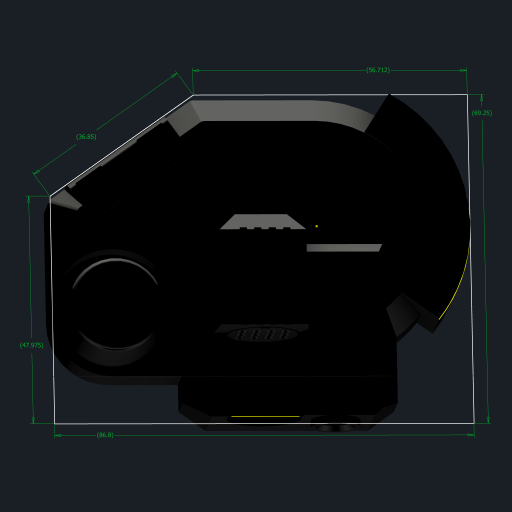
# Autodesk Inventor part: MidiController
Saved by Autodesk Inventor 2023 (Build 270158000, 158)
## iProperties
Created: 2023-06-16
Part Number: MidiController
Material: Generic
Document SubType Name: Modeling
Designer: valer
Density: 1 g/cm^3
Appearance: Default
Author: valer
Autodesk Inventor part; units mm, degrees
ref_plane "YZ Plane" through (0, 0, 0) normal (1, 0, 0) x (0, 1, 0)
ref_plane "XZ Plane" through (0, 0, 0) normal (0, 1, 0) x (-1, 0, 0)
ref_plane "XY Plane" through (0, 0, 0) normal (0, 0, 1) x (1, 0, 0)
sketch "Sketch1" plane through (0, 0, 0) normal (0, 0, 1) x (1, 0, 0)
  line L0 (-41.4, 33.875) -> (41.4, 33.875) construction
  line L1 (41.4, 33.875) -> (41.4, -33.875) construction
  line L2 (41.4, -33.875) -> (-41.4, -33.875) construction
  line L3 (-41.4, -33.875) -> (-41.4, 33.875) construction
  line L4 (-59.3343, 0) -> (66.206, 0) construction
  line L5 (0, -48.6206) -> (0, 54.5983) construction
  circle A0 centre (-28.595, -11.3999) radius 10.805 construction
  circle A1 centre (-28.595, -11.3999) radius 12.805
  line L6 (-28.595, -24.2049) -> (-14.35, -24.2049)
  line L7 (-14.35, -24.2049) -> (-14.35, -29.875)
  line L8 (-14.35, -29.875) -> (-8.85, -33.875)
  line L9 (-8.85, -33.875) -> (24.75, -33.875)
  line L10 (24.75, -33.875) -> (30.25, -29.875)
  line L11 (30.25, -29.875) -> (30.25, -16.055)
  line L12 (-14.35, -29.875) -> (30.25, -29.875) construction
  line L13 (-41.4, -11.3999) -> (-41.4, 12.6001)
  line L14 (-11.3118, 33.875) -> (-41.4, 12.6001)
  arc A2 (30.25, -16.055) -> (13.6882, 33.875) centre (13.6882, 6.1632) ccw
  line L15 (-11.3118, 33.875) -> (13.6882, 33.875)
  point P0 (0, 0)
  point P1 (-41.4, 0)
  point P2 (0, 33.875)
  dimension "d0" = 82.8
  dimension "d1" = 67.75
  dimension "d2" = 21.61
  dimension "d3" = 2
  dimension "d4" = 44.6
  dimension "d5" = 4
  dimension "d6" = 5.5
  dimension "d7" = 11.15
  dimension "d9" = 36.85
  dimension "d10" = 24
  dimension "d11" = 25
  dimension "d12" = 13.82
  constraints: 28 end point, 8 point on line, 5 tangent, 4 point on circle, 3 centre point, 3 perpendicular, 2 horizontal, 2 midpoint, 2 parallel, 1 coincident, 1 collinear, 1 equal length, 1 vertical
  measures "d0" distance of L0.start L0.end
  measures "d1" distance of L2.end L0.start
  measures "d2" diameter of A0
  measures "d3" radial gap between concentric circles of A1 A0
  measures "d4" distance between parallel lines of L11 L7
  measures "d5" distance between parallel lines of L9 L12
  measures "d6" horizontal distance of L7.end L8.end
  measures "d7" distance between parallel lines of L1 L11
  measures "d9" distance of L14.start L13.end
  measures "d10" distance of L13.start L13.end
  measures "d11" distance of L15.end L14.start
  measures "d12" distance of L10.end L11.end
extrude "Extrusion1" add sketch "Sketch1" along normal blind 9
sketch "Sketch2" plane through (0, 0, 9) normal (0, 0, 1) x (1, 0, 0)
  line L0 (-14.35, -29.875) -> (-8.85, -33.875) projected
  line L1 (-8.85, -33.875) -> (24.75, -33.875) projected
  line L2 (24.75, -33.875) -> (30.25, -29.875) projected
  line L3 (30.25, -29.875) -> (30.25, -16.055) projected
  arc A0 (30.25, -16.055) -> (13.6882, 33.875) centre (13.6882, 6.1632) ccw projected
  line L4 (13.6882, 33.875) -> (-11.3118, 33.875) projected
  line L5 (-11.3118, 33.875) -> (-41.4, 12.6001) projected
  line L6 (-41.4, 12.6001) -> (-41.4, -11.3999) projected
  arc A1 (-41.4, -11.3999) -> (-28.595, -24.2049) centre (-28.595, -11.3999) ccw projected
  line L7 (-28.595, -24.2049) -> (-14.35, -24.2049) projected
  line L8 (-14.35, -24.2049) -> (-14.35, -29.875) projected
  point P0 (0, 0)
extrude "Extrusion2" add sketch "Sketch2" along normal blind 5.5 draft -45
sketch "Sketch4" plane through (0, 0, 14.5) normal (0, 0, 1) x (1, 0, 0)
  circle A0 centre (-28.595, -11.3999) radius 10.805
  arc A1 (-41.4, -11.3999) -> (-28.595, -24.2049) centre (-28.595, -11.3999) ccw projected
  line L0 (-41.4, -11.3999) -> (-35.9, -11.3999) projected
  circle A2 centre (-28.595, -11.3999) radius 12.805
  point P0 (0, 0)
  dimension "d18" = 21.61
  constraints: 1 centre point, 1 coincident, 1 concentric, 3 other
  measures "d18" diameter of A0
extrude "Extrusion3" cut sketch "Sketch4" against normal up to surface (5.5 mm away) contours A0 | A2 A1
sketch "Sketch5" plane through (-28.595, -11.3999, 9) normal (0, 0, 1) x (0.7071068, 0.7071068, 0)
  arc A0 (-9.0545, -9.0545) -> (-9.0545, 9.0545) centre (0, 0) ccw construction
  arc A1 (-9.0545, 9.0545) -> (-9.0545, -9.0545) centre (0, 0) ccw construction
  circle A2 centre (0, 0) radius 10.805
  point P0 (28.2807, -12.1588)
  dimension "d21" = 21.61
  constraints: 1 centre point, 1 coincident
  measures "d21" diameter of A2
extrude "Extrusion4" add sketch "Sketch5" along normal blind 11.4 draft -5
fillet "Fillet1" radius 2 2 edges at (-41.4, 12.6001, 4.5) (-11.3118, 33.875, 4.5)
fillet "Fillet2" radius 2 2 edges at (-38.5381, 11.1186, 11.8619) (-10.4228, 31.078, 11.797)
fillet "Fillet4" radius 1 1 edges at (-35.53, -18.3349, 20.4)
sketch "Sketch7" plane through (-8.85, -33.875, 0) normal (0, -1, 0) x (1, 0, 0)
  line L0 (39.1, 17.83) -> (-5.5, 17.83) construction
  line L1 (-5.5, 17.83) -> (-5.5, 0) construction
  line L2 (-5.5, 0) -> (39.1, 0) construction
  line L3 (39.1, 0) -> (39.1, 17.83) construction
  line L4 (0, 0) -> (33.6, 0) projected
  line L5 (39.1, 0) -> (39.1, 9) projected
  line L6 (-5.5, 0) -> (-5.5, 9) projected
  line L7 (39.1, 9) -> (34.9825, 17.83)
  line L8 (34.9825, 17.83) -> (20.1325, 17.83)
  line L9 (20.1325, 17.83) -> (18.5797, 14.5)
  line L10 (-0.2642, 14.5) -> (22.5382, 14.5) construction
  circle A0 centre (11.0964, 12.3) radius 7.8 construction
  line L11 (-5.5, 0) -> (-5.5, 9) projected
  line L12 (-5.5, 4.5) -> (39.1, 4.5) construction
  line L13 (1.7885, 14.5) -> (0, 14.5) projected
  line L14 (3.6131, 14.5) -> (0, 14.5)
  line L15 (0, 14.5) -> (-5.5, 9)
  line L16 (39.1, 9) -> (-5.5, 9)
  line L17 (-2.9808, 9) -> (-31.7047, 9) projected
  arc A1 (3.6131, 14.5) -> (18.5797, 14.5) centre (11.0964, 12.3) ccw
  line L18 (-5.5, 0) -> (39.1, 0)
  line L19 (50.25, 0) -> (22.5382, 0) projected
  line L20 (39.1, 9) -> (39.1, 0)
  line L21 (-19.745, 9) -> (-5.5, 9) projected
  line L22 (-5.5, 9) -> (-5.5, 0)
  point P0 (8.85, 0)
  dimension "d28" = 17.83
  dimension "d29" = 14.85
  dimension "d31" = 115
  dimension "d32" = 115
  dimension "d33" = 15.6
  constraints: 28 end point, 7 collinear, 4 point on circle, 4 point on line, 2 centre point, 2 concentric, 2 horizontal, 2 midpoint, 2 parallel, 1 perpendicular, 1 tangent
  measures "d28" distance of L2.end L0.start
  measures "d29" distance of L7.end L8.end
  measures "d31" angle of L0 L7
  measures "d32" angle of L0 L9
  measures "d33" diameter of A0
sketch "Sketch8" plane through (0, 0, 0) normal (0, 0, -1) x (-1, 0, 0)
  line L0 (14.35, -29.875) -> (8.85, -33.875) projected
  line L1 (14.35, -29.875) -> (8.85, -33.875)
  line L2 (8.85, -33.875) -> (14.35, -33.875)
  line L3 (14.35, -33.875) -> (14.35, -29.875)
  line L4 (-24.75, -33.875) -> (-30.25, -29.875) projected
  line L5 (-30.25, -29.875) -> (-24.75, -33.875)
  line L6 (-24.75, -33.875) -> (-30.25, -33.875)
  line L7 (-30.25, -33.875) -> (-30.25, -29.875)
  line L8 (-30.25, -29.875) -> (-30.25, -16.055) projected
  line L9 (8.85, -33.875) -> (-24.75, -33.875) projected
  point P0 (0, 0)
  constraints: 12 end point, 4 collinear, 2 horizontal, 2 perpendicular
extrude "Extrusion5" add sketch "Sketch7" against normal blind 36 contours L18 L6 L16 A1 L5 L4 | L15 L13 L14 A1 L16 | L16 A1 L9 L8 L7
extrude "Extrusion6" cut sketch "Sketch8" against normal blind 36
sketch "Sketch9" plane through (-4.8211, -33.875, 9) normal (0, -1, 0) x (1, 0, 0)
  line L0 (14.5508, 5.5) -> (-0.4158, 5.5) projected
  circle A0 centre (7.0675, 3.3708) radius 7.7803
  point P0 (4.8211, -9)
  constraints: 3 other
extrude "Extrusion7" cut sketch "Sketch9" against normal blind 17.67
sketch "Sketch10" plane through (-4.8211, -16.205, 9) normal (0, -1, 0) x (1, 0, 0)
  line L0 (16.1037, 8.83) -> (30.9537, 8.83) projected
  line L1 (16.1037, 8.83) -> (15.576, 13.85)
  line L2 (15.576, 13.85) -> (-2.3696, 13.85)
  line L3 (-2.3696, 13.85) -> (-3.2472, 5.5)
  line L4 (-0.4158, 5.5) -> (-4.0289, 5.5) projected
  arc A0 (14.1351, 0) -> (14.5508, 5.5) centre (7.0675, 3.3) ccw projected
  line L5 (-3.2472, 5.5) -> (14.5508, 5.5)
  line L6 (14.5508, 5.5) -> (16.1037, 8.83) projected
  line L7 (14.5508, 5.5) -> (16.1037, 8.83)
  line L8 (-4.0289, -9) -> (29.5711, -9) projected
  point P0 (4.8211, -9)
  dimension "d40" = 22.85
  dimension "d41" = 96
  dimension "d42" = 96
  constraints: 10 end point, 1 collinear, 1 horizontal, 1 parallel, 1 point on line
  measures "d40" distance between parallel lines of L8 L2
  measures "d41" angle of L2 L1
  measures "d42" angle of L2 L3
extrude "Extrusion8" add sketch "Sketch10" against normal blind 20
sketch "Sketch11" plane through (-4.8211, 3.795, 9) normal (0, 1, 0) x (1, 0, 0)
  line L0 (-3.2472, -5.5) -> (-2.3696, -13.85) projected
  line L1 (-2.3696, -13.85) -> (15.576, -13.85) projected
  line L2 (15.576, -13.85) -> (16.1037, -8.83) projected
  line L3 (16.1037, -8.83) -> (14.5508, -5.5) projected
  line L4 (-3.2472, -5.5) -> (14.5508, -5.5) projected
  point P0 (4.8211, 9)
extrude "Extrusion9" add sketch "Sketch11" along normal blind 4 separate body
chamfer "Chamfer1" distance 4 angle 45 2 edges at (-7.6296, 7.795, 18.675) (11.0187, 7.795, 20.34)
chamfer "Chamfer2" distance 4 angle 45 1 edges at (1.7821, 7.795, 22.85)
chamfer "Chamfer3" distance 2 angle 45 1 edges at (18.7075, 2.125, 17.83)
combine bodies "Combine1" operation type add bodies to combine 1 2
sketch "Sketch12" plane through (-4.8211, -16.205, 9) normal (0, -1, 0) x (1, 0, 0)
  arc A0 (0.0553, 0) -> (14.0798, 0) centre (7.0675, 3.3708) ccw projected
  arc A1 (-0.4158, 5.5) -> (0, 0) centre (7.0675, 3.3) ccw projected
  circle A2 centre (7.0675, 3.3708) radius 7.8302
  point P0 (4.8211, -9)
  constraints: 1 coincident, 3 other
extrude "Extrusion10" cut sketch "Sketch12" against normal blind 6 bodies 1
sketch "Sketch13" plane through (2.2464, -10.205, 12.3708) normal (0, -1, 0) x (1, 0, 0)
  circle A0 centre (0, 0) radius 7.8302 projected
  circle A1 centre (0, 0) radius 7.3302
  point P0 (-2.2464, -12.3708)
  dimension "d59" = 0.5
  constraints: 1 centre point, 1 coincident
  measures "d59" radial gap between concentric circles of A0 A1
extrude "Extrusion11" add sketch "Sketch13" along normal blind 6 contours A1 bodies 1
sketch "Sketch14" plane through (2.2464, -16.205, 12.3708) normal (0, -1, 0) x (1, 0, 0)
  circle A0 centre (0, 0) radius 7.3302 construction
  line L0 (0, 0) -> (0, -7.3302)
  line L1 (11.4418, -3.3708) -> (-12.9225, -3.3708) construction
  line L2 (-1, 7.3302) -> (1, 7.3302)
  line L3 (1, 7.3302) -> (1, 6.3302)
  line L4 (1, 6.3302) -> (-1, 6.3302)
  line L5 (-1, 6.3302) -> (-1, 7.3302)
  line L6 (8.5085, 10.4792) -> (-9.4372, 10.4792) construction
  line L7 (0, 0) -> (0, 10.4792) construction
  point P0 (-2.2464, -12.3708)
  point P1 (-12.9225, -3.3708)
  point P2 (0, 6.3302)
  dimension "d62" = 2
  dimension "d63" = 1
  constraints: 12 end point, 2 horizontal, 2 parallel, 2 point on line, 2 vertical, 1 midpoint, 1 perpendicular, 1 vertical alignment, 2 other
  measures "d62" distance of L3.end L4.end
  measures "d63" distance between parallel lines of L4 L2
extrude "Extrusion12" cut sketch "Sketch14" against normal blind 6 bodies 1
sketch "Sketch15" plane through (2.2464, -16.205, 12.3708) normal (0, -1, 0) x (1, 0, 0)
  line L0 (-4.5, 3) -> (4.5, 3) construction
  line L1 (4.5, 3) -> (4.5, -3) construction
  line L2 (4.5, -3) -> (-4.5, -3) construction
  line L3 (-4.5, -3) -> (-4.5, 3) construction
  line L4 (-4.5, 0) -> (4.5, 0) construction
  line L5 (9.0361, 5.4592) -> (8.5085, 10.4792) projected
  arc A0 (-1, 7.2617) -> (1, 7.2617) centre (0, 0) ccw projected
  line L6 (-1.5, 3) -> (-1.5, -3) construction
  line L7 (1.5, 3) -> (1.5, -3) construction
  circle A1 centre (-4.5, 3) radius 0.75
  circle A2 centre (-1.5, 3) radius 0.75
  circle A3 centre (1.5, 3) radius 0.75
  circle A4 centre (4.5, 3) radius 0.75
  circle A5 centre (-4.5, 0) radius 0.75
  circle A6 centre (-1.5, 0) radius 0.75
  circle A7 centre (1.5, 0) radius 0.75
  circle A8 centre (4.5, 0) radius 0.75
  circle A9 centre (4.5, -3) radius 0.75
  circle A10 centre (1.5, -3) radius 0.75
  circle A11 centre (-1.5, -3) radius 0.75
  circle A12 centre (-4.5, -3) radius 0.75
  point P0 (-2.2464, -12.3708)
  dimension "d66" = 9
  dimension "d69" = 6
  dimension "d70" = 1.5
  dimension "d71" = 3
  dimension "d72" = 3
  constraints: 14 end point, 12 centre point, 11 coincident, 11 equal radius, 5 midpoint, 4 point on line, 3 perpendicular, 2 parallel, 1 horizontal
  measures "d66" distance of L0.start L0.end
  measures "d69" distance of L2.end L0.start
  measures "d70" diameter of A1
  measures "d71" distance between parallel lines of L3 L6
  measures "d72" distance between parallel lines of L1 L7
extrude "Extrusion13" cut sketch "Sketch15" against normal blind 6 bodies 1
chamfer "Chamfer4" distance 0.5 angle 45 12 edges at (-3.0036, -16.205, 15.3708) (-0.0036, -16.205, 15.3708) (2.9964, -16.205, 15.3708) (5.9964, -16.205, 15.3708) (5.9964, -16.205, 12.3708) (2.9964, -16.205, 12.3708) (-0.0036, -16.205, 12.3708) (-3.0036, -16.205, 12.3708) (-3.0036, -16.205, 9.3708) (-0.0036, -16.205, 9.3708) (2.9964, -16.205, 9.3708) (5.9964, -16.205, 9.3708)
chamfer "Chamfer5" distance 2 angle 45 1 edges at (18.0163, -33.875, 17.83)
sketch "Sketch17" plane through (-8.85, -33.875, 0) normal (0, -1, 0) x (1, 0, 0)
  circle A0 centre (25.965, 10.695) radius 5.135
  line L0 (19.1999, 15.83) -> (33.6, 15.83) construction
  line L1 (33.6, 0) -> (33.6, 15.83) projected
  point P0 (8.85, 0)
  dimension "d81" = 10.27
  dimension "d82" = 7.635
  constraints: 1 centre point, 1 tangent
  measures "d81" diameter of A0
  measures "d82" distance from line of L1 A0.centre
extrude "Extrusion14" add sketch "Sketch17" along normal blind 1.5 bodies 1
sketch "Sketch18" plane through (17.115, -35.375, 10.695) normal (0, -1, 0) x (1, 0, 0)
  circle A0 centre (0, 0) radius 5.135 projected
  circle A1 centre (0, 0) radius 3.2
  point P0 (-17.115, -10.695)
  dimension "d86" = 6.4
  constraints: 1 centre point, 1 coincident
  measures "d86" diameter of A1
extrude "Extrusion15" cut sketch "Sketch18" against normal blind 10 contours A1 bodies 1
chamfer "Chamfer6" distance 1 angle 45 1 edges at (13.915, -35.375, 10.695)
sketch "Sketch19" plane through (0, 0, 0) normal (0, 0, -1) x (-1, 0, 0)
  arc A0 (-13.6882, 33.875) -> (-30.25, -16.055) centre (-13.6882, 6.1632) ccw projected
  arc A1 (-13.6882, 37.875) -> (-32.6406, -19.262) centre (-13.6882, 6.1632) ccw
  line L0 (-29.1056, 33.875) -> (-26.9244, 30.5096)
  arc A2 (-13.6882, 33.875) -> (-30.25, -16.055) centre (-13.6882, 6.1632) ccw projected
  line L1 (-38.5813, -13.4829) -> (-35.3393, -11.1335)
  point P0 (0, 0)
  dimension "d92" = 4
  constraints: 6 point on circle, 4 end point, 1 centre point
  measures "d92" radial gap between concentric circles of A0 A1
extrude "Extrusion16" add sketch "Sketch19" against normal blind 15.5 bodies 1
sketch "Sketch20" plane through (0, 0, 15.5) normal (0, 0, 1) x (1, 0, 0)
  line L0 (35.3393, -11.1335) -> (38.5813, -13.4829) projected
  line L1 (38.5813, -13.4829) -> (30.8795, -7.9017)
  arc A0 (27.6853, -11.0833) -> (13.6882, 28.375) centre (13.6882, 6.1632) ccw projected
  line L2 (29.1056, 33.875) -> (23.9219, 25.877)
  line L3 (29.1056, 33.875) -> (26.9244, 30.5096) projected
  arc A1 (38.5813, -13.4829) -> (29.1056, 33.875) centre (13.6882, 6.1632) ccw projected
  point P0 (0, 0)
  constraints: 4 end point, 2 collinear, 2 point on circle
extrude "Extrusion17" add sketch "Sketch20" against normal up to surface (15.5 mm away) bodies 1
sketch "Sketch21" plane through (0, 0, 14.5) normal (0, 0, 1) x (1, 0, 0)
  line L0 (-37.851, 15.1095) -> (-17.4384, 29.543)
  line L1 (-17.4384, 29.543) -> (-10.7758, 20.1204)
  line L2 (-10.7758, 20.1204) -> (-31.1884, 5.6869)
  line L3 (-31.1884, 5.6869) -> (-37.851, 15.1095)
  line L4 (-11.8308, 33.508) -> (-40.5547, 13.1978) projected
  ellipse E0 centre (-33.0716, 8.2889) end of major axis (-35.7464, 9.6735) minor radius 2 (-35.3023, 10.1757) -> (-35.9, 9.021) ccw projected
  point P0 (0, 0)
  dimension "d98" = 25
  constraints: 8 end point, 2 collinear, 2 parallel, 1 perpendicular, 1 other
  measures "d98" distance of L1.end L2.end
extrude "Extrusion18" add sketch "Sketch21" against normal up to surface (14.5 mm away) bodies 1
fillet "Fillet6" radius 1.5 1 edges at (-27.6447, 22.3263, 14.5)
sketch "Sketch22" plane through (0, 0, 14.5) normal (0, 0, 1) x (1, 0, 0)
  line L0 (-36.0489, 15.159) -> (-30.8641, 18.8251)
  line L1 (-30.8641, 18.8251) -> (-25.9856, 11.9257)
  line L2 (-25.9856, 11.9257) -> (-31.1704, 8.2596)
  line L3 (-31.1704, 8.2596) -> (-36.0489, 15.159)
  line L4 (-17.4384, 29.543) -> (-37.851, 15.1095) projected
  line L5 (-27.6447, 22.3263) -> (-22.1888, 14.6103) construction
  line L6 (-25.9856, 11.9257) -> (-22.1888, 14.6103) construction
  line L7 (-36.985, 13.8848) -> (-34.6757, 10.6188) projected
  line L8 (-18.0858, 27.8605) -> (-23.2706, 24.1944)
  line L9 (-23.2706, 24.1944) -> (-18.3921, 17.2949)
  line L10 (-18.3921, 17.2949) -> (-13.2073, 20.961)
  line L11 (-13.2073, 20.961) -> (-18.0858, 27.8605)
  point P0 (0, 0)
  point P1 (-35.8303, 12.2518)
  dimension "d102" = 1
  dimension "d103" = 8.45
  dimension "d104" = 1.5
  dimension "d105" = 6.35
  constraints: 20 end point, 4 symmetric about line, 3 parallel, 3 perpendicular, 2 midpoint
  measures "d102" distance between parallel lines of L4 L0
  measures "d103" distance of L2.end L0.start
  measures "d104" distance from line of L3 point (-35.83, 12.252)
  measures "d105" distance of L1.end L2.end
extrude "Extrusion19" add sketch "Sketch22" along normal blind 1 bodies 1
sketch "Sketch23" plane through (-7.1908, -16.205, 22.85) normal (0, 0, 1) x (1, 0, 0)
  line L0 (5.6872, 0.5) -> (4.1872, 0.5) construction
  line L1 (8.6872, 0.5) -> (7.1872, 0.5) construction
  line L2 (11.6872, 0.5) -> (10.1872, 0.5) construction
  line L3 (14.6872, 0.5) -> (13.1872, 0.5) construction
  line L4 (17.9456, 0) -> (0, 0) construction
  line L5 (4.9372, 0) -> (4.9372, 20) construction
  line L6 (0, 20) -> (17.9456, 20) construction
  line L7 (7.9372, 0) -> (7.9372, 20) construction
  line L8 (10.9372, 0) -> (10.9372, 20) construction
  line L9 (13.9372, 0) -> (13.9372, 20) construction
  line L10 (4.1872, 20) -> (5.6872, 20)
  line L11 (5.6872, 20) -> (5.6872, 0)
  line L12 (5.6872, 0) -> (4.1872, 0)
  line L13 (4.1872, 0) -> (4.1872, 20)
  line L14 (7.1872, 0) -> (8.6872, 0)
  line L15 (8.6872, 0) -> (8.6872, 20)
  line L16 (8.6872, 20) -> (7.1872, 20)
  line L17 (7.1872, 20) -> (7.1872, 0)
  line L18 (8.9728, 0) -> (8.9728, 20) construction
  line L19 (10.1872, 20) -> (11.6872, 20)
  line L20 (11.6872, 20) -> (11.6872, 0)
  line L21 (11.6872, 0) -> (10.1872, 0)
  line L22 (10.1872, 0) -> (10.1872, 20)
  line L23 (13.1872, 20) -> (14.6872, 20)
  line L24 (14.6872, 20) -> (14.6872, 0)
  line L25 (14.6872, 0) -> (13.1872, 0)
  line L26 (13.1872, 0) -> (13.1872, 20)
  point P0 (7.1908, 16.205)
  point P1 (4.9372, 0.5)
  point P2 (7.9372, 0.5)
  point P3 (10.9372, 0.5)
  point P4 (13.9372, 0.5)
  point P5 (10.9372, 20)
  point P6 (13.9372, 20)
  constraints: 42 end point, 9 parallel, 8 horizontal, 8 point on line, 7 midpoint, 4 perpendicular, 3 collinear, 3 vertical, 17 other
extrude "Extrusion20" cut sketch "Sketch23" against normal blind 0.5 bodies 1
delete faces "Delete1" heal yes whole lump no faces at (-2.0036, 3.795, 22.5167) (0.9964, 3.795, 22.5167) (3.9964, 3.795, 22.6833) (6.9964, 3.795, 22.6833)
fillet "Fillet7" radius 0.125 16 edges at (-1.5036, -5.9549, 22.35) (-1.5036, -6.205, 22.85) (-3.0036, -5.9549, 22.35) (-3.0036, -6.205, 22.85) (-0.0036, -6.205, 22.85) (-0.0036, -5.9549, 22.35) (1.4964, -5.9549, 22.35) (1.4964, -6.205, 22.85) (2.9964, -6.205, 22.85) (4.4964, -6.205, 22.85) (4.4964, -5.9549, 22.35) (5.9964, -6.205, 22.85) (7.4964, -6.205, 22.85) (7.4964, -5.9549, 22.35) (2.9964, -5.9549, 22.35) (5.9964, -5.9549, 22.35)
sketch "Sketch24" plane through (0, 0, 14.5) normal (0, 0, 1) x (1, 0, 0)
  line L0 (-41.4, 11.5648) -> (-41.4, -11.3999) projected
  line L1 (13.6882, 33.875) -> (-10.6761, 33.875) projected
  arc A0 (38.5813, -13.4829) -> (29.1056, 33.875) centre (13.6882, 6.1632) ccw projected
  line L2 (9.2586, -33.875) -> (-4.7659, -33.875) projected
  line L3 (11.98, -35.375) -> (22.25, -35.375) projected
  line L4 (-41.4, 12.6001) -> (-41.4, -35.375)
  line L5 (-41.4, -35.375) -> (45.4, -35.375)
  line L6 (45.4, -35.375) -> (45.4, 33.875)
  line L7 (45.4, 33.875) -> (-11.3118, 33.875)
  line L8 (-11.3118, 33.875) -> (-41.4, 12.6001)
  line L9 (-17.4384, 29.543) -> (-37.851, 15.1095) projected
  line L10 (-11.8308, 33.508) -> (-17.4384, 29.543) projected
  point P0 (0, 0)
  dimension "d111" = 36.85
  dimension "d112" = 56.7118
  dimension "d113" = 47.9751
  dimension "d114" = 86.8
  dimension "d115" = 69.25
  constraints: 10 end point, 5 collinear, 3 perpendicular, 1 tangent, 1 vertical
  measures "d111" distance of L7.end L4.start
  measures "d112" distance of L6.end L7.end
  measures "d113" distance of L4.start L4.end
  measures "d114" distance of L4.end L5.end
  measures "d115" distance of L5.end L6.end
equation "\"d32\" = d31"
equation "\"d42\" = d41"
equation "\"d71\" = 0.333333 * d66"
equation "\"d72\" = 0.333333 * d66"
body "Solid1"
